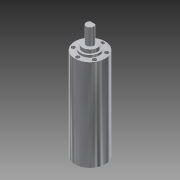
# Autodesk Inventor part: Motor
Saved by Autodesk Inventor 2015 (Build 190159000, 159)
## iProperties
Created: 2016-09-19
Part Number: Motor
Material: Generic
Document SubType Name: Modeling
Designer: James Yelland
Density: 1 g/cm^3
Appearance: Default
Author: James Yelland
Autodesk Inventor part; units mm, degrees
ref_plane "XZ Plane" through (0, 0, 0) normal (0, 1, 0) x (-1, 0, 0)
ref_plane "XY Plane" through (0, 0, 0) normal (0, 0, 1) x (1, 0, 0)
sketch "Sketch1" plane through (0, 0, 0) normal (0, 0, 1) x (1, 0, 0)
  circle A0 centre (0, 0) radius 8
  dimension "d0" = 16
  constraints: 1 centre point, 1 coincident
  measures "d0" diameter of A0
extrude "Extrusion1" add sketch "Sketch1" along normal blind 48.6
sketch "Sketch2" plane through (0, 0, 48.6) normal (0, 0, 1) x (1, 0, 0)
  circle A0 centre (0, 6.5) radius 1
  circle A1 centre (5.6292, 3.25) radius 1
  circle A2 centre (5.6292, -3.25) radius 1
  circle A3 centre (0, -6.5) radius 1
  circle A4 centre (-5.6292, -3.25) radius 1
  circle A5 centre (-5.6292, 3.25) radius 1
  point P0 (0, 0)
  point P1 (0, 0)
  dimension "d5" = 2
  dimension "d8" = 360
  constraints: 6 centre point, 13 other
  measures "d5" diameter of A0
extrude "Extrusion2" cut sketch "Sketch2" against normal blind 10
sketch "Sketch3" plane through (0, 0, 48.6) normal (0, 0, 1) x (1, 0, 0)
  circle A0 centre (0, 0) radius 5
  dimension "d12" = 10
  constraints: 1 centre point, 1 coincident
  measures "d12" diameter of A0
extrude "Extrusion3" add sketch "Sketch3" along normal blind 1.15
sketch "Sketch4" plane through (0, 0, 49.75) normal (0, 0, 1) x (1, 0, 0)
  circle A0 centre (0, 0) radius 4
  dimension "d15" = 8
  constraints: 1 centre point, 1 coincident
  measures "d15" diameter of A0
extrude "Extrusion4" add sketch "Sketch4" along normal blind 1.85
sketch "Sketch5" plane through (0, 0, 51.6) normal (0, 0, 1) x (1, 0, 0)
  circle A0 centre (0, 0) radius 2
  dimension "d18" = 4
  constraints: 1 centre point, 1 coincident
  measures "d18" diameter of A0
extrude "Extrusion5" add sketch "Sketch5" along normal blind 8.75
sketch "Sketch6" plane through (0, 0, 60.35) normal (0, 0, 1) x (1, 0, 0)
  circle A0 centre (0, 0) radius 2
  circle A1 centre (0, 0) radius 2 projected
  line L0 (0, 2) -> (0, 1.5)
  line L1 (0, 1.5) -> (-1.3229, 1.5)
  line L2 (0, 1.5) -> (1.3229, 1.5)
  line L3 (0, 1.5) -> (1.3229, 1.5) construction
  dimension "d23" = 0.5
  dimension "d24" = 90
  dimension "d25" = 0
  constraints: 8 end point, 3 point on circle, 1 centre point, 1 collinear, 1 horizontal, 1 vertical
  measures "d23" distance of L0.start L0.end
  measures "d24" angle of L0 L1
  measures "d25" distance between parallel lines of L2 L3
extrude "Extrusion6" cut sketch "Sketch6" against normal blind 8 contours L2 L0 A0 | A0 L0 L1
ref_plane "Work Plane1" through (2, 0, 51.6) normal (1, 0, 0) x (0, 1, 0)
sketch "Sketch7" plane through (2, 0, 51.6) normal (1, 0, 0) x (0, 1, 0)
  line L0 (-2, 0) -> (2, 0) projected
  line L1 (1.5, 8.75) -> (1.5, 0.75) projected
  line L2 (1.5, 0.75) -> (1.5, 0.75) projected
  line L3 (1.5, 0.75) -> (1.5, 8.75) projected
  line L4 (1.5, 8.75) -> (1.5, 8.75) projected
  line L5 (2, 0) -> (2, 0.2)
  line L6 (2, 0.2) -> (1.5, 0.75)
  line L7 (2, 0.75) -> (1.5, 0.75)
  line L8 (2, 0.75) -> (2, 0.2)
  point P0 (0, -51.6)
  dimension "d30" = 0.2
  constraints: 8 end point, 2 perpendicular, 1 vertical
  measures "d30" distance of L0.end L5.end
extrude "Extrusion7" cut sketch "Sketch7" against normal through all
body "Solid1"
